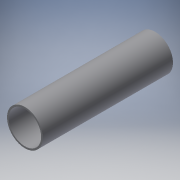
# Autodesk Inventor part: pipe_110mm_0.75m
Saved by Autodesk Inventor 2017 (Build 210142000, 142)
## iProperties
Created: 2014-08-21
Part Number: pipe_110mm_0.75m
Material: Generic
Document SubType Name: Modeling
Designer: Dave
Density: 1 g/cm^3
Appearance: Default
Author: Dave
Autodesk Inventor part; units mm, degrees
ref_plane "YZ Plane" through (0, 0, 0) normal (1, 0, 0) x (0, 1, 0)
ref_plane "XZ Plane" through (0, 0, 0) normal (0, 1, 0) x (-1, 0, 0)
ref_plane "XY Plane" through (0, 0, 0) normal (0, 0, 1) x (1, 0, 0)
sketch "Sketch1" plane through (0, 0, 0) normal (0, 0, 1) x (1, 0, 0)
  circle A0 centre (0.1401, 0) radius 55
  circle A1 centre (0.1401, 0) radius 49.92
  point P0 (0, 0)
  dimension "d1" = 5.08
  dimension "d2" = 110
  constraints: 2 centre point
  measures "d1" radial gap between concentric circles of A1 A0
  measures "d2" diameter of A0
extrude "Extrusion1" add sketch "Sketch1" along normal blind 300
body "Solid1"
